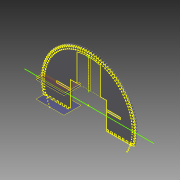
# Autodesk Inventor part: Spur Gear2
Saved by Autodesk Inventor 2013 (Build 170138000, 138)
## iProperties
Created: 2013-02-22
Part Number: Spur Gear2
Material: Steel
Document SubType Name: Modeling
Designer: Nano
Categories: <?xml version="1.0" encoding="UTF-16"?> <MemberInstance><Categories><FamilyTemplate><FamilyTemplateParameter ValueType="xs:double" Id="1" ObjectReferenceKey="da_z" ObjectType="kUserParameterObject"/><FamilyTemplateParameter ValueType="xs:double" Id="2" ObjectReferenceKey="da_b" ObjectType="kUserParameterObject"/><FamilyTemplateParameter ValueType="xs:double" Id="3" ObjectReferenceKey="da_beta" ObjectType="kUserParameterObject"/><FamilyTemplateParameter ValueType="xs:double" Id="4" ObjectReferenceKey="da_da" ObjectType="kUserParameterObject"/><FamilyTemplateParameter ValueType="xs:double" Id="5" ObjectReferenceKey="da_aw" ObjectType="kUserParameterObject"/><FamilyTemplateParameter ValueType="xs:string" Id="6" ObjectReferenceKey="EAIAABAAAAC/AAAAAAAAAIAAAAAAAAAA" ObjectType="83910656" SubObjectId="SurfaceGeometry"/></FamilyTemplate><ParamToTemplateMap><ParamToTemplate CategoryParameter="//CategoryParameter[@InternalName='046C89C9-8512-4d59-83FE-43B91F4F132A']" TemplateParameter="1"/><ParamToTemplate CategoryParameter="//CategoryParameter[@InternalName='2552DF32-E462-4b46-AEBF-C6C7768E72AC']" TemplateParameter="2"/><ParamToTemplate CategoryParameter="//CategoryParameter[@InternalName='C9EE641D-15FC-4fae-A226-E94C4372FDD7']" TemplateParameter="3"/><ParamToTemplate><ParamToTemplate CategoryParameter="//CategoryParameter[@InternalName='00B6519A-459B-49c7-AD84-2E56D39A5744']" ConstantValue="0.000000"/></ParamToTemplate><ParamToTemplate><ParamToTemplate CategoryParameter="//CategoryParameter[@InternalName='04B31F0E-C7A6-4894-AA32-9629BEFACF47']" ConstantValue="1.000000"/></ParamToTemplate><ParamToTemplate><ParamToTemplate CategoryParameter="//CategoryParameter[@InternalName='43CBEC2E-7847-49e7-A936-2F7889FCB2D9']" ConstantValue="0.250000"/></ParamToTemplate><ParamToTemplate><ParamToTemplate CategoryParameter="//CategoryParameter[@InternalName='B1EFC894-105D-4ebd-86BF-FA20ED196853']" ConstantValue="0.350000"/></ParamToTemplate><ParamToTemplate><ParamToTemplate CategoryParameter="//CategoryParameter[@InternalName='51175063-3D10-4879-93E8-6246FE8B403D']" ConstantValue="2060110000.000000"/></ParamToTemplate><ParamToTemplate><ParamToTemplate CategoryParameter="//CategoryParameter[@InternalName='A3A52E27-4454-46a9-B0BD-C932399B70AF']" ConstantValue="0.300000"/></ParamToTemplate><ParamToTemplate><ParamToTemplate CategoryParameter="//CategoryParameter[@InternalName='91B76062-C214-41d9-B1B9-14D2AB99603D']" ConstantValue="0.254000"/></ParamToTemplate><ParamToTemplate><ParamToTemplate CategoryParameter="//CategoryParameter[@InternalName='374E806E-8B8A-4dda-A9AA-1039D6500AD2']" ConstantValue="3.937008"/></ParamToTemplate><ParamToTemplate><ParamToTemplate CategoryParameter="//CategoryParameter[@InternalName='2D373A89-B862-43d6-8D0B-0CBF12AB9F6C']" ConstantValue="0.349066"/></ParamToTemplate><ParamToTemplate CategoryParameter="//CategoryParameter[@InternalName='37777632-D6A2-4fac-9D53-DB8ACD95C989']" TemplateParameter="4"/><ParamToTemplate CategoryParameter="//CategoryParameter[@InternalName='FD1017F1-B727-4f7e-9707-0F86F1FF9423']" TemplateParameter="5"/><ParamToTemplate><ParamToTemplate CategoryParameter="//CategoryParameter[@InternalName='9E1B4470-B2D3-4ff1-B813-535BB4CDF51A']" ConstantValue="3520790.000000"/></ParamToTemplate><ParamToTemplate><ParamToTemplate CategoryParameter="//CategoryParameter[@InternalName='F8452263-BFF6-458c-9FB1-07C4B99E95CD']" ConstantValue="11389170.000000"/></ParamToTemplate><ParamToTemplate><ParamToTemplate CategoryParameter="//CategoryParameter[@InternalName='3E3BB259-FD49-497f-8171-6EBC954A3479']" ConstantValue="2.000000"/></ParamToTemplate><ParamToTemplate CategoryParameter="//CategoryParameter[@InternalName='27C3BAF2-7550-4e4b-AE2C-0DB134B7D9B7']" TemplateParameter="6"/></ParamToTemplateMap><Category DisplayName="Gear" InternalName="DC85795E-93AB-48d5-8EEE-5A27447B64BD" Mnemonic="Gear"><CategoryParameter DisplayName="z" InternalName="046C89C9-8512-4d59-83FE-43B91F4F132A" Mnemonic="z"/><CategoryParameter DisplayName="b" InternalName="2552DF32-E462-4b46-AEBF-C6C7768E72AC" Mnemonic="b"/><CategoryParameter DisplayName="||b|" InternalName="C9EE641D-15FC-4fae-A226-E94C4372FDD7" Mnemonic="beta"/><CategoryParameter DisplayName="x" InternalName="00B6519A-459B-49c7-AD84-2E56D39A5744" Mnemonic="x"/><CategoryParameter DisplayName="a*" InternalName="04B31F0E-C7A6-4894-AA32-9629BEFACF47" Mnemonic="a"/><CategoryParameter DisplayName="c*" InternalName="43CBEC2E-7847-49e7-A936-2F7889FCB2D9" Mnemonic="c"/><CategoryParameter DisplayName="r|.f|*" InternalName="B1EFC894-105D-4ebd-86BF-FA20ED196853" Mnemonic="rf"/><CategoryParameter DisplayName="E" InternalName="51175063-3D10-4879-93E8-6246FE8B403D" Mnemonic="E"/><CategoryParameter DisplayName="||m|" InternalName="A3A52E27-4454-46a9-B0BD-C932399B70AF" Mnemonic="mi"/><Category DisplayName="SpurGear" InternalName="26C5A22E-A91E-4dfd-A3B3-23CCAFAE1764" Mnemonic="SpurGear"><CategoryParameter DisplayName="m" InternalName="91B76062-C214-41d9-B1B9-14D2AB99603D" Mnemonic="m"/><CategoryParameter DisplayName="P" InternalName="374E806E-8B8A-4dda-A9AA-1039D6500AD2" Mnemonic="PP"/><CategoryParameter DisplayName="||a|" InternalName="2D373A89-B862-43d6-8D0B-0CBF12AB9F6C" Mnemonic="alpha"/><CategoryParameter DisplayName="d|.a|" InternalName="37777632-D6A2-4fac-9D53-DB8ACD95C989" Mnemonic="da"/><CategoryParameter DisplayName="a|.w|" InternalName="FD1017F1-B727-4f7e-9707-0F86F1FF9423" Mnemonic="aw"/><CategoryParameter DisplayName="||s||.Flim|" InternalName="9E1B4470-B2D3-4ff1-B813-535BB4CDF51A" Mnemonic="sFlim"/><CategoryParameter DisplayName="||s||.Hlim|" InternalName="F8452263-BFF6-458c-9FB1-07C4B99E95CD" Mnemonic="sHlim"/><CategoryParameter DisplayName="type" InternalName="3E3BB259-FD49-497f-8171-6EBC954A3479" Mnemonic="type"/><CategoryParameter DisplayName="PitchDiameter" InternalName="27C3BAF2-7550-4e4b-AE2C-0DB134B7D9B7" Mnemonic="IDS_PITCHDIAM"/></Category></Category></Categories></MemberInstance>
Density: 1 g/cm^3
CustomPartVersion: 1
Author: Nano
Autodesk Inventor part; units mm, degrees
(part 1 of 2)
ref_plane "YZ Plane" through (0, 0, 0) normal (1, 0, 0) x (0, 1, 0)
ref_plane "XZ Plane" through (0, 0, 0) normal (0, 1, 0) x (-1, 0, 0)
ref_plane "XY Plane" through (0, 0, 0) normal (0, 0, 1) x (1, 0, 0)
sketch "Sketch1" plane through (0, 0, 0) normal (0, 0, 1) x (1, 0, 0)
  circle A0 centre (0, 0) radius 154.94
  dimension "d0" = 309.88
  constraints: 1 centre point
  measures "d0" diameter of A0
extrude "Extrusion1" add sketch "Sketch1" along normal blind 6.35
sketch "Sketch2" plane through (0, 0, 0) normal (0, 0, -1) x (-1, 0, 0)
  circle A0 centre (0, 0) radius 154.94 projected
  circle A1 centre (0, 0) radius 152.4
  dimension "d3" = 304.8
  constraints: 1 centre point, 1 coincident
  measures "d3" diameter of A1
surface extrude "Pitch Diameter" sketch "Sketch2" against normal through all shown no curves A1
ref_plane "Work Plane1" through (0, 0, 0) normal (1, 0, 0) x (0, 1, 0)
ref_plane "Work Plane2" through (0, 0, 0) normal (0.9996573, 0.0261769, 0) x (0, 0, 1)
ref_plane "Work Plane3" through (0, 0, 3.175) normal (0, 0, -1) x (-1, 0, 0)
spur gear teeth "Spur Gear" teeth 120 pitch diameter 304.8 tip diameter 309.88 root diameter 298.45 face width 6.35 start plane through (0, 0, 0) normal (0, 0, -1) x (-1, 0, 0)
sketch "Sketch3" plane through (0, 0, 6.35) normal (0, 0, 1) x (1, 0, 0)
  line L0 (-226.2292, -43.1165) -> (223.5893, -43.1165)
  constraints: 2 end point
split body "Split1" sketch "Sketch3" result one side removed curves L0 removed pieces at (21.5954, -83.6344, 0.5)
sketch "Sketch4" plane through (0, 0, 6.35) normal (0, 0, 1) x (1, 0, 0)
  line L0 (-142.8603, -43.1165) -> (142.8603, -43.1165) projected
  line L1 (-59.5312, -44.45) -> (59.5312, -44.45)
  line L2 (59.5312, -44.45) -> (59.5312, 44.45)
  line L3 (59.5312, 44.45) -> (38.1, 44.45)
  line L4 (-59.5312, 44.45) -> (-59.5312, -44.45)
  line L5 (-59.5312, -44.45) -> (59.5312, 44.45) construction
  line L6 (59.5312, -44.45) -> (-59.5312, 44.45) construction
  line L7 (-38.1, -3.175) -> (38.1, -3.175)
  line L8 (38.1, -3.175) -> (38.1, 133.985)
  line L9 (38.1, 133.985) -> (-38.1, 133.985)
  line L10 (-38.1, 133.985) -> (-38.1, -3.175)
  line L11 (-38.1, -3.175) -> (38.1, 133.985) construction
  line L12 (38.1, -3.175) -> (-38.1, 133.985) construction
  arc A0 (-133.0152, -43.1165) -> (38.1, 133.985) centre (0, -0.4192) ccw
  arc A1 (-38.1, 133.985) -> (-133.0152, -43.1165) centre (0, -0.4192) ccw
  arc A2 (38.1, 133.985) -> (-38.1, 133.985) centre (0, -0.4192) ccw
  line L13 (-38.1, 44.45) -> (-59.5312, 44.45)
  line L14 (38.1, 44.45) -> (-38.1, 44.45)
  point P0 (0, 0)
  point P1 (0, 65.405)
  dimension "d20" = 119.0625
  dimension "d21" = 88.9
  dimension "d22" = 76.2
  dimension "d23" = 137.16
  dimension "d24" = 279.4
  constraints: 28 end point, 6 parallel, 6 point on circle, 4 midpoint, 3 centre point, 3 point on line, 2 perpendicular
  measures "d20" distance of L1.start L1.end
  measures "d21" distance of L2.end L1.end
  measures "d22" distance of L7.start L7.end
  measures "d23" distance of L8.end L7.end
  measures "d24" diameter of A0
extrude "Extrusion2" cut sketch "Sketch4" against normal through all contours L4 L13 L10 L7 L8 L3 L2 L0 | L0 L2 L1 L4 | A2 L9 | L9 L8 L14 L10 | L14 L8 L7 L10
ref_plane "Work Plane4" through (-93.1308, -43.1165, 3.175) normal (0, -1, 0) x (1, 0, 0)
sketch "Sketch5" plane through (-93.1308, -43.1165, 3.175) normal (0, -1, 0) x (1, 0, 0)
  line L0 (-36.2504, 3.175) -> (-36.2504, -3.175) projected
  line L1 (-36.2504, -3.175) -> (-42.6004, -3.175) projected
  line L2 (-42.6004, -3.175) -> (-42.6004, 3.175) projected
  line L3 (-42.6004, 3.175) -> (-36.2504, 3.175) projected
  line L4 (-23.5504, 3.175) -> (-23.5504, -3.175) projected
  line L5 (-23.5504, -3.175) -> (-29.9004, -3.175) projected
  line L6 (-29.9004, -3.175) -> (-29.9004, 3.175) projected
  line L7 (-29.9004, 3.175) -> (-23.5504, 3.175) projected
  line L8 (-10.8504, 3.175) -> (-10.8504, -3.175) projected
  line L9 (-10.8504, -3.175) -> (-17.2004, -3.175) projected
  line L10 (-17.2004, -3.175) -> (-17.2004, 3.175) projected
  line L11 (-17.2004, 3.175) -> (-10.8504, 3.175) projected
  line L12 (1.8496, 3.175) -> (1.8496, -3.175) projected
  line L13 (1.8496, -3.175) -> (-4.5004, -3.175) projected
  line L14 (-4.5004, -3.175) -> (-4.5004, 3.175) projected
  line L15 (-4.5004, 3.175) -> (1.8496, 3.175) projected
  line L16 (14.5496, 3.175) -> (14.5496, -3.175) projected
  line L17 (14.5496, -3.175) -> (8.1996, -3.175) projected
  line L18 (8.1996, -3.175) -> (8.1996, 3.175) projected
  line L19 (8.1996, 3.175) -> (14.5496, 3.175) projected
  line L20 (27.2496, 3.175) -> (27.2496, -3.175) projected
  line L21 (27.2496, -3.175) -> (20.8996, -3.175) projected
  line L22 (20.8996, -3.175) -> (20.8996, 3.175) projected
  line L23 (20.8996, 3.175) -> (27.2496, 3.175) projected
  line L24 (-49.7295, -3.175) -> (33.5996, -25.4) projected
  line L25 (33.5996, -25.4) -> (33.5996, 25.4) projected
  line L26 (33.5996, 25.4) -> (-49.7295, 3.175) projected
  line L27 (-49.7295, 3.175) -> (-49.7295, -3.175) projected
  point P0 (93.1308, -3.175)
extrude "Extrusion3" cut sketch "Sketch5" against normal blind 6.35
sketch "Sketch6" plane through (0, 0, 6.35) normal (0, 0, 1) x (1, 0, 0)
  line L0 (-65.8813, -36.7665) -> (-59.5312, -36.7665) projected
  line L1 (-59.5312, -36.7665) -> (-59.5312, 44.45) projected
  line L2 (-59.5312, 44.45) -> (-38.1, 44.45) projected
  line L3 (-38.1, 44.45) -> (-38.1, 133.985) projected
  arc A0 (38.1, 133.985) -> (-38.1, 133.985) centre (0, -0.4192) ccw projected
  line L4 (38.1, 133.985) -> (38.1, 44.45) projected
  line L5 (38.1, 44.45) -> (59.5312, 44.45) projected
  line L6 (59.5312, 44.45) -> (59.5312, -43.1165) projected
  line L7 (59.5312, -43.1165) -> (142.8603, -43.1165) projected
  arc A1 (142.8603, -43.1165) -> (143.3542, -41.4448) centre (0, 0) ccw projected
  arc A2 (143.3542, -41.4448) -> (149.3949, -41.0801) centre (144.1598, -4.5833) ccw projected
  arc A3 (149.3949, -41.0801) -> (149.9198, -39.121) centre (0, 0) ccw projected
  arc A4 (149.9198, -39.121) -> (144.8708, -35.7848) centre (127.1377, -68.1106) ccw projected
  arc A5 (144.8708, -35.7848) -> (145.3268, -33.8855) centre (0, 0) ccw projected
  arc A6 (145.3268, -33.8855) -> (151.3401, -33.2051) centre (144.2021, 2.9677) ccw projected
  arc A7 (151.3401, -33.2051) -> (151.7618, -31.2212) centre (0, 0) ccw projected
  arc A8 (151.7618, -31.2212) -> (146.5451, -28.1538) centre (130.5281, -61.3634) ccw projected
  arc A9 (146.5451, -28.1538) -> (146.9011, -26.2332) centre (0, 0) ccw projected
  arc A10 (146.9011, -26.2332) -> (152.8705, -25.239) centre (143.8491, 10.5106) ccw projected
  arc A11 (152.8705, -25.239) -> (153.1878, -23.2358) centre (0, 0) ccw projected
  arc A12 (153.1878, -23.2358) -> (147.8177, -20.4457) centre (133.5607, -54.448) ccw projected
  arc A13 (147.8177, -20.4457) -> (148.0727, -18.509) centre (0, 0) ccw projected
  arc A14 (148.0727, -18.509) -> (153.9819, -17.2038) centre (143.1019, 18.0247) ccw projected
  arc A15 (153.9819, -17.2038) -> (154.1939, -15.1868) centre (0, 0) ccw projected
  arc A16 (154.1939, -15.1868) -> (148.6852, -12.6815) centre (136.2272, -47.3834) ccw projected
  arc A17 (148.6852, -12.6815) -> (148.8384, -10.7342) centre (0, 0) ccw projected
  arc A18 (148.8384, -10.7342) -> (154.6713, -9.1214) centre (141.9624, 25.4894) ccw projected
  arc A19 (154.6713, -9.1214) -> (154.7774, -7.0961) centre (0, 0) ccw projected
  arc A20 (154.7774, -7.0961) -> (149.1451, -4.8825) centre (138.5204, -40.1889) ccw projected
  arc A21 (149.1451, -4.8825) -> (149.1962, -2.9298) centre (0, 0) ccw projected
  arc A22 (149.1962, -2.9298) -> (154.9367, -1.0141) centre (140.4339, 32.8842) ccw projected
  arc A23 (154.9367, -1.0141) -> (154.9367, 1.0141) centre (0, 0) ccw projected
  arc A24 (154.9367, 1.0141) -> (149.1962, 2.9298) centre (140.4339, -32.8842) ccw projected
  arc A25 (149.1962, 2.9298) -> (149.1451, 4.8825) centre (0, 0) ccw projected
  arc A26 (149.1451, 4.8825) -> (154.7774, 7.0961) centre (138.5204, 40.1889) ccw projected
  arc A27 (154.7774, 7.0961) -> (154.6713, 9.1214) centre (0, 0) ccw projected
  arc A28 (154.6713, 9.1214) -> (148.8384, 10.7342) centre (141.9624, -25.4894) ccw projected
  arc A29 (148.8384, 10.7342) -> (148.6852, 12.6815) centre (0, 0) ccw projected
  arc A30 (148.6852, 12.6815) -> (154.1939, 15.1868) centre (136.2272, 47.3834) ccw projected
  arc A31 (154.1939, 15.1868) -> (153.9819, 17.2038) centre (0, 0) ccw projected
  arc A32 (153.9819, 17.2038) -> (148.0727, 18.509) centre (143.1019, -18.0247) ccw projected
  arc A33 (148.0727, 18.509) -> (147.8177, 20.4457) centre (0, 0) ccw projected
  arc A34 (147.8177, 20.4457) -> (153.1878, 23.2358) centre (133.5607, 54.448) ccw projected
  arc A35 (153.1878, 23.2358) -> (152.8705, 25.239) centre (0, 0) ccw projected
  arc A36 (152.8705, 25.239) -> (146.9011, 26.2332) centre (143.8491, -10.5106) ccw projected
  arc A37 (146.9011, 26.2332) -> (146.5451, 28.1538) centre (0, 0) ccw projected
  arc A38 (146.5451, 28.1538) -> (151.7618, 31.2212) centre (130.5281, 61.3634) ccw projected
  arc A39 (151.7618, 31.2212) -> (151.3401, 33.2051) centre (0, 0) ccw projected
  arc A40 (151.3401, 33.2051) -> (145.3268, 33.8855) centre (144.2021, -2.9677) ccw projected
  arc A41 (145.3268, 33.8855) -> (144.8708, 35.7848) centre (0, 0) ccw projected
  arc A42 (144.8708, 35.7848) -> (149.9198, 39.121) centre (127.1377, 68.1106) ccw projected
  arc A43 (149.9198, 39.121) -> (149.3949, 41.0801) centre (0, 0) ccw projected
  arc A44 (149.3949, 41.0801) -> (143.3542, 41.4448) centre (144.1598, 4.5833) ccw projected
  arc A45 (143.3542, 41.4448) -> (142.7994, 43.3177) centre (0, 0) ccw projected
  arc A46 (142.7994, 43.3177) -> (147.6669, 46.9136) centre (123.3988, 74.6712) ccw projected
  arc A47 (147.6669, 46.9136) -> (147.0402, 48.8425) centre (0, 0) ccw projected
  arc A48 (147.0402, 48.8425) -> (140.9887, 48.8906) centre (143.7223, 12.1217) ccw projected
  arc A49 (140.9887, 48.8906) -> (140.3366, 50.7319) centre (0, 0) ccw projected
  arc A50 (140.3366, 50.7319) -> (145.0093, 54.5776) centre (119.3217, 81.027) ccw projected
  arc A51 (145.0093, 54.5776) -> (144.2824, 56.4711) centre (0, 0) ccw projected
  arc A52 (144.2824, 56.4711) -> (138.2367, 56.2024) centre (142.891, 19.627) ccw projected
  arc A53 (138.2367, 56.2024) -> (137.4892, 58.007) centre (0, 0) ccw projected
  arc A54 (137.4892, 58.007) -> (141.9542, 62.092) centre (114.9175, 87.1608) ccw projected
  arc A55 (141.9542, 62.092) -> (141.1292, 63.9448) centre (0, 0) ccw projected
  arc A56 (141.1292, 63.9448) -> (135.1059, 63.3601) centre (141.6679, 27.0784) ccw projected
  arc A57 (135.1059, 63.3601) -> (134.2649, 65.1232) centre (0, 0) ccw projected
  arc A58 (134.2649, 65.1232) -> (138.51, 69.4362) centre (110.1984, 93.0557) ccw projected
  arc A59 (138.51, 69.4362) -> (137.5892, 71.2433) centre (0, 0) ccw projected
  arc A60 (137.5892, 71.2433) -> (131.6047, 70.3442) centre (140.0566, 34.4556) ccw projected
  arc A61 (131.6047, 70.3442) -> (130.6726, 72.0608) centre (0, 0) ccw projected
  arc A62 (130.6726, 72.0608) -> (134.6861, 76.5901) centre (105.1772, 98.6955) ccw projected
  arc A63 (134.6861, 76.5901) -> (133.6721, 78.3466) centre (0, 0) ccw projected
  arc A64 (133.6721, 78.3466) -> (127.7428, 77.1354) centre (138.0614, 41.7384) ccw projected
  arc A65 (127.7428, 77.1354) -> (126.7222, 78.8009) centre (0, 0) ccw projected
  arc A66 (126.7222, 78.8009) -> (130.4931, 83.5341) centre (99.8678, 104.0648) ccw projected
  arc A67 (130.4931, 83.5341) -> (129.3885, 85.235) centre (0, 0) ccw projected
  arc A68 (129.3885, 85.235) -> (123.5308, 83.7153) centre (135.6878, 48.9068) ccw projected
  arc A69 (123.5308, 83.7153) -> (122.4244, 85.3251) centre (0, 0) ccw projected
  arc A70 (122.4244, 85.3251) -> (125.9425, 90.2491) centre (94.2846, 109.1488) ccw projected
  arc A71 (125.9425, 90.2491) -> (124.7504, 91.8899) centre (0, 0) ccw projected
  arc A72 (124.7504, 91.8899) -> (118.9802, 90.0656) centre (132.9422, 55.9411) ccw projected
  arc A73 (118.9802, 90.0656) -> (117.7911, 91.6153) centre (0, 0) ccw projected
  arc A74 (117.7911, 91.6153) -> (121.0466, 96.7167) centre (88.4429, 113.9337) ccw projected
  arc A75 (121.0466, 96.7167) -> (119.7702, 98.2929) centre (0, 0) ccw projected
  arc A76 (119.7702, 98.2929) -> (114.1034, 96.1691) centre (129.8323, 62.8221) ccw projected
  arc A77 (114.1034, 96.1691) -> (112.8349, 97.6545) centre (0, 0) ccw projected
  arc A78 (112.8349, 97.6545) -> (115.8189, 102.9193) centre (82.3589, 118.4063) ccw projected
  arc A79 (115.8189, 102.9193) -> (114.4618, 104.4265) centre (0, 0) ccw projected
  arc A80 (114.4618, 104.4265) -> (108.914, 102.0091) centre (126.3665, 69.5309) ccw projected
  arc A81 (108.914, 102.0091) -> (107.5694, 103.426) centre (0, 0) ccw projected
  arc A82 (107.5694, 103.426) -> (110.2738, 108.8397) centre (76.0491, 122.5544) ccw projected
  arc A83 (110.2738, 108.8397) -> (108.8397, 110.2738) centre (0, 0) ccw projected
  arc A84 (108.8397, 110.2738) -> (103.426, 107.5694) centre (122.5544, 76.0491) ccw projected
  arc A85 (103.426, 107.5694) -> (102.0091, 108.914) centre (0, 0) ccw projected
  arc A86 (102.0091, 108.914) -> (104.4265, 114.4618) centre (69.5309, 126.3665) ccw projected
  arc A87 (104.4265, 114.4618) -> (102.9193, 115.8189) centre (0, 0) ccw projected
  arc A88 (102.9193, 115.8189) -> (97.6545, 112.8349) centre (118.4063, 82.3589) ccw projected
  arc A89 (97.6545, 112.8349) -> (96.1691, 114.1034) centre (0, 0) ccw projected
  arc A90 (96.1691, 114.1034) -> (98.2929, 119.7702) centre (62.8221, 129.8323) ccw projected
  arc A91 (98.2929, 119.7702) -> (96.7167, 121.0466) centre (0, 0) ccw projected
  arc A92 (96.7167, 121.0466) -> (91.6153, 117.7911) centre (113.9337, 88.4429) ccw projected
  arc A93 (91.6153, 117.7911) -> (90.0656, 118.9802) centre (0, 0) ccw projected
  arc A94 (90.0656, 118.9802) -> (91.8899, 124.7504) centre (55.9411, 132.9422) ccw projected
  arc A95 (91.8899, 124.7504) -> (90.2491, 125.9425) centre (0, 0) ccw projected
  arc A96 (90.2491, 125.9425) -> (85.3251, 122.4244) centre (109.1488, 94.2846) ccw projected
  arc A97 (85.3251, 122.4244) -> (83.7153, 123.5308) centre (0, 0) ccw projected
  arc A98 (83.7153, 123.5308) -> (85.235, 129.3885) centre (48.9068, 135.6878) ccw projected
  arc A99 (85.235, 129.3885) -> (83.5341, 130.4931) centre (0, 0) ccw projected
  arc A100 (83.5341, 130.4931) -> (78.8009, 126.7222) centre (104.0648, 99.8678) ccw projected
  arc A101 (78.8009, 126.7222) -> (77.1354, 127.7428) centre (0, 0) ccw projected
  arc A102 (77.1354, 127.7428) -> (78.3466, 133.6721) centre (41.7384, 138.0614) ccw projected
  arc A103 (78.3466, 133.6721) -> (76.5901, 134.6861) centre (0, 0) ccw projected
  arc A104 (76.5901, 134.6861) -> (72.0608, 130.6726) centre (98.6955, 105.1772) ccw projected
  arc A105 (72.0608, 130.6726) -> (70.3442, 131.6047) centre (0, 0) ccw projected
  arc A106 (70.3442, 131.6047) -> (71.2433, 137.5892) centre (34.4556, 140.0566) ccw projected
  arc A107 (71.2433, 137.5892) -> (69.4362, 138.51) centre (0, 0) ccw projected
  arc A108 (69.4362, 138.51) -> (65.1232, 134.2649) centre (93.0557, 110.1984) ccw projected
  arc A109 (65.1232, 134.2649) -> (63.3601, 135.1059) centre (0, 0) ccw projected
  arc A110 (63.3601, 135.1059) -> (63.9448, 141.1292) centre (27.0784, 141.6679) ccw projected
  arc A111 (63.9448, 141.1292) -> (62.092, 141.9542) centre (0, 0) ccw projected
  arc A112 (62.092, 141.9542) -> (58.007, 137.4892) centre (87.1608, 114.9175) ccw projected
  arc A113 (58.007, 137.4892) -> (56.2024, 138.2367) centre (0, 0) ccw projected
  arc A114 (56.2024, 138.2367) -> (56.4711, 144.2824) centre (19.627, 142.891) ccw projected
  arc A115 (56.4711, 144.2824) -> (54.5776, 145.0093) centre (0, 0) ccw projected
  arc A116 (54.5776, 145.0093) -> (50.7319, 140.3366) centre (81.027, 119.3217) ccw projected
  arc A117 (50.7319, 140.3366) -> (48.8906, 140.9887) centre (0, 0) ccw projected
  arc A118 (48.8906, 140.9887) -> (48.8425, 147.0402) centre (12.1217, 143.7223) ccw projected
  arc A119 (48.8425, 147.0402) -> (46.9136, 147.6669) centre (0, 0) ccw projected
  arc A120 (46.9136, 147.6669) -> (43.3177, 142.7994) centre (74.6712, 123.3988) ccw projected
  arc A121 (43.3177, 142.7994) -> (41.4448, 143.3542) centre (0, 0) ccw projected
  arc A122 (41.4448, 143.3542) -> (41.0801, 149.3949) centre (4.5833, 144.1598) ccw projected
  arc A123 (41.0801, 149.3949) -> (39.121, 149.9198) centre (0, 0) ccw projected
  arc A124 (39.121, 149.9198) -> (35.7848, 144.8708) centre (68.1106, 127.1377) ccw projected
  arc A125 (35.7848, 144.8708) -> (33.8855, 145.3268) centre (0, 0) ccw projected
  arc A126 (33.8855, 145.3268) -> (33.2051, 151.3401) centre (-2.9677, 144.2021) ccw projected
  arc A127 (33.2051, 151.3401) -> (31.2212, 151.7618) centre (0, 0) ccw projected
  arc A128 (31.2212, 151.7618) -> (28.1538, 146.5451) centre (61.3634, 130.5281) ccw projected
  arc A129 (28.1538, 146.5451) -> (26.2332, 146.9011) centre (0, 0) ccw projected
  arc A130 (26.2332, 146.9011) -> (25.239, 152.8705) centre (-10.5106, 143.8491) ccw projected
  arc A131 (25.239, 152.8705) -> (23.2358, 153.1878) centre (0, 0) ccw projected
  arc A132 (23.2358, 153.1878) -> (20.4457, 147.8177) centre (54.448, 133.5607) ccw projected
  arc A133 (20.4457, 147.8177) -> (18.509, 148.0727) centre (0, 0) ccw projected
  arc A134 (18.509, 148.0727) -> (17.2038, 153.9819) centre (-18.0247, 143.1019) ccw projected
  arc A135 (17.2038, 153.9819) -> (15.1868, 154.1939) centre (0, 0) ccw projected
  arc A136 (15.1868, 154.1939) -> (12.6815, 148.6852) centre (47.3834, 136.2272) ccw projected
  arc A137 (12.6815, 148.6852) -> (10.7342, 148.8384) centre (0, 0) ccw projected
  arc A138 (10.7342, 148.8384) -> (9.1214, 154.6713) centre (-25.4894, 141.9624) ccw projected
  arc A139 (9.1214, 154.6713) -> (7.0961, 154.7774) centre (0, 0) ccw projected
  arc A140 (7.0961, 154.7774) -> (4.8825, 149.1451) centre (40.1889, 138.5204) ccw projected
  arc A141 (4.8825, 149.1451) -> (2.9298, 149.1962) centre (0, 0) ccw projected
  arc A142 (2.9298, 149.1962) -> (1.0141, 154.9367) centre (-32.8842, 140.4339) ccw projected
  arc A143 (1.0141, 154.9367) -> (-1.0141, 154.9367) centre (0, 0) ccw projected
  arc A144 (-1.0141, 154.9367) -> (-2.9298, 149.1962) centre (32.8842, 140.4339) ccw projected
  arc A145 (-2.9298, 149.1962) -> (-4.8825, 149.1451) centre (0, 0) ccw projected
  arc A146 (-4.8825, 149.1451) -> (-7.0961, 154.7774) centre (-40.1889, 138.5204) ccw projected
  arc A147 (-7.0961, 154.7774) -> (-9.1214, 154.6713) centre (0, 0) ccw projected
  arc A148 (-9.1214, 154.6713) -> (-10.7342, 148.8384) centre (25.4894, 141.9624) ccw projected
  arc A149 (-10.7342, 148.8384) -> (-12.6815, 148.6852) centre (0, 0) ccw projected
  arc A150 (-12.6815, 148.6852) -> (-15.1868, 154.1939) centre (-47.3834, 136.2272) ccw projected
  arc A151 (-15.1868, 154.1939) -> (-17.2038, 153.9819) centre (0, 0) ccw projected
  arc A152 (-17.2038, 153.9819) -> (-18.509, 148.0727) centre (18.0247, 143.1019) ccw projected
  arc A153 (-18.509, 148.0727) -> (-20.4457, 147.8177) centre (0, 0) ccw projected
  arc A154 (-20.4457, 147.8177) -> (-23.2358, 153.1878) centre (-54.448, 133.5607) ccw projected
  arc A155 (-23.2358, 153.1878) -> (-25.239, 152.8705) centre (0, 0) ccw projected
  arc A156 (-25.239, 152.8705) -> (-26.2332, 146.9011) centre (10.5106, 143.8491) ccw projected
  arc A157 (-26.2332, 146.9011) -> (-28.1538, 146.5451) centre (0, 0) ccw projected
  arc A158 (-28.1538, 146.5451) -> (-31.2212, 151.7618) centre (-61.3634, 130.5281) ccw projected
  arc A159 (-31.2212, 151.7618) -> (-33.2051, 151.3401) centre (0, 0) ccw projected
  arc A160 (-33.2051, 151.3401) -> (-33.8855, 145.3268) centre (2.9677, 144.2021) ccw projected
  arc A161 (-33.8855, 145.3268) -> (-35.7848, 144.8708) centre (0, 0) ccw projected
  arc A162 (-35.7848, 144.8708) -> (-39.121, 149.9198) centre (-68.1106, 127.1377) ccw projected
  arc A163 (-39.121, 149.9198) -> (-41.0801, 149.3949) centre (0, 0) ccw projected
  arc A164 (-41.0801, 149.3949) -> (-41.4448, 143.3542) centre (-4.5833, 144.1598) ccw projected
  arc A165 (-41.4448, 143.3542) -> (-43.3177, 142.7994) centre (0, 0) ccw projected
  arc A166 (-43.3177, 142.7994) -> (-46.9136, 147.6669) centre (-74.6712, 123.3988) ccw projected
  arc A167 (-46.9136, 147.6669) -> (-48.8425, 147.0402) centre (0, 0) ccw projected
  arc A168 (-48.8425, 147.0402) -> (-48.8906, 140.9887) centre (-12.1217, 143.7223) ccw projected
  arc A169 (-48.8906, 140.9887) -> (-50.7319, 140.3366) centre (0, 0) ccw projected
  arc A170 (-50.7319, 140.3366) -> (-54.5776, 145.0093) centre (-81.027, 119.3217) ccw projected
  arc A171 (-54.5776, 145.0093) -> (-56.4711, 144.2824) centre (0, 0) ccw projected
  arc A172 (-56.4711, 144.2824) -> (-56.2024, 138.2367) centre (-19.627, 142.891) ccw projected
  arc A173 (-56.2024, 138.2367) -> (-58.007, 137.4892) centre (0, 0) ccw projected
  arc A174 (-58.007, 137.4892) -> (-62.092, 141.9542) centre (-87.1608, 114.9175) ccw projected
  arc A175 (-62.092, 141.9542) -> (-63.9448, 141.1292) centre (0, 0) ccw projected
  arc A176 (-63.9448, 141.1292) -> (-63.3601, 135.1059) centre (-27.0784, 141.6679) ccw projected
  arc A177 (-63.3601, 135.1059) -> (-65.1232, 134.2649) centre (0, 0) ccw projected
  arc A178 (-65.1232, 134.2649) -> (-69.4362, 138.51) centre (-93.0557, 110.1984) ccw projected
  arc A179 (-69.4362, 138.51) -> (-71.2433, 137.5892) centre (0, 0) ccw projected
  arc A180 (-71.2433, 137.5892) -> (-70.3442, 131.6047) centre (-34.4556, 140.0566) ccw projected
  arc A181 (-70.3442, 131.6047) -> (-72.0608, 130.6726) centre (0, 0) ccw projected
  arc A182 (-72.0608, 130.6726) -> (-76.5901, 134.6861) centre (-98.6955, 105.1772) ccw projected
  arc A183 (-76.5901, 134.6861) -> (-78.3466, 133.6721) centre (0, 0) ccw projected
  arc A184 (-78.3466, 133.6721) -> (-77.1354, 127.7428) centre (-41.7384, 138.0614) ccw projected
  arc A185 (-77.1354, 127.7428) -> (-78.8009, 126.7222) centre (0, 0) ccw projected
  arc A186 (-78.8009, 126.7222) -> (-83.5341, 130.4931) centre (-104.0648, 99.8678) ccw projected
  arc A187 (-83.5341, 130.4931) -> (-85.235, 129.3885) centre (0, 0) ccw projected
  arc A188 (-85.235, 129.3885) -> (-83.7153, 123.5308) centre (-48.9068, 135.6878) ccw projected
  arc A189 (-83.7153, 123.5308) -> (-85.3251, 122.4244) centre (0, 0) ccw projected
  arc A190 (-85.3251, 122.4244) -> (-90.2491, 125.9425) centre (-109.1488, 94.2846) ccw projected
  arc A191 (-90.2491, 125.9425) -> (-91.8899, 124.7504) centre (0, 0) ccw projected
  arc A192 (-91.8899, 124.7504) -> (-90.0656, 118.9802) centre (-55.9411, 132.9422) ccw projected
  arc A193 (-90.0656, 118.9802) -> (-91.6153, 117.7911) centre (0, 0) ccw projected
  arc A194 (-91.6153, 117.7911) -> (-96.7167, 121.0466) centre (-113.9337, 88.4429) ccw projected
  arc A195 (-96.7167, 121.0466) -> (-98.2929, 119.7702) centre (0, 0) ccw projected
  arc A196 (-98.2929, 119.7702) -> (-96.1691, 114.1034) centre (-62.8221, 129.8323) ccw projected
  arc A197 (-96.1691, 114.1034) -> (-97.6545, 112.8349) centre (0, 0) ccw projected
  arc A198 (-97.6545, 112.8349) -> (-102.9193, 115.8189) centre (-118.4063, 82.3589) ccw projected
  arc A199 (-102.9193, 115.8189) -> (-104.4265, 114.4618) centre (0, 0) ccw projected
  arc A200 (-104.4265, 114.4618) -> (-102.0091, 108.914) centre (-69.5309, 126.3665) ccw projected
  arc A201 (-102.0091, 108.914) -> (-103.426, 107.5694) centre (0, 0) ccw projected
  arc A202 (-103.426, 107.5694) -> (-108.8397, 110.2738) centre (-122.5544, 76.0491) ccw projected
  arc A203 (-108.8397, 110.2738) -> (-110.2738, 108.8397) centre (0, 0) ccw projected
  arc A204 (-110.2738, 108.8397) -> (-107.5694, 103.426) centre (-76.0491, 122.5544) ccw projected
  arc A205 (-107.5694, 103.426) -> (-108.914, 102.0091) centre (0, 0) ccw projected
  arc A206 (-108.914, 102.0091) -> (-114.4618, 104.4265) centre (-126.3665, 69.5309) ccw projected
  arc A207 (-114.4618, 104.4265) -> (-115.8189, 102.9193) centre (0, 0) ccw projected
  arc A208 (-115.8189, 102.9193) -> (-112.8349, 97.6545) centre (-82.3589, 118.4063) ccw projected
  arc A209 (-112.8349, 97.6545) -> (-114.1034, 96.1691) centre (0, 0) ccw projected
  arc A210 (-114.1034, 96.1691) -> (-119.7702, 98.2929) centre (-129.8323, 62.8221) ccw projected
  arc A211 (-119.7702, 98.2929) -> (-121.0466, 96.7167) centre (0, 0) ccw projected
  arc A212 (-121.0466, 96.7167) -> (-117.7911, 91.6153) centre (-88.4429, 113.9337) ccw projected
  arc A213 (-117.7911, 91.6153) -> (-118.9802, 90.0656) centre (0, 0) ccw projected
  arc A214 (-118.9802, 90.0656) -> (-124.7504, 91.8899) centre (-132.9422, 55.9411) ccw projected
  arc A215 (-124.7504, 91.8899) -> (-125.9425, 90.2491) centre (0, 0) ccw projected
  arc A216 (-125.9425, 90.2491) -> (-122.4244, 85.3251) centre (-94.2846, 109.1488) ccw projected
  arc A217 (-122.4244, 85.3251) -> (-123.5308, 83.7153) centre (0, 0) ccw projected
  arc A218 (-123.5308, 83.7153) -> (-129.3885, 85.235) centre (-135.6878, 48.9068) ccw projected
  arc A219 (-129.3885, 85.235) -> (-130.4931, 83.5341) centre (0, 0) ccw projected
  arc A220 (-130.4931, 83.5341) -> (-126.7222, 78.8009) centre (-99.8678, 104.0648) ccw projected
  arc A221 (-126.7222, 78.8009) -> (-127.7428, 77.1354) centre (0, 0) ccw projected
  arc A222 (-127.7428, 77.1354) -> (-133.6721, 78.3466) centre (-138.0614, 41.7384) ccw projected
  arc A223 (-133.6721, 78.3466) -> (-134.6861, 76.5901) centre (0, 0) ccw projected
  arc A224 (-134.6861, 76.5901) -> (-130.6726, 72.0608) centre (-105.1772, 98.6955) ccw projected
  arc A225 (-130.6726, 72.0608) -> (-131.6047, 70.3442) centre (0, 0) ccw projected
  arc A226 (-131.6047, 70.3442) -> (-137.5892, 71.2433) centre (-140.0566, 34.4556) ccw projected
  arc A227 (-137.5892, 71.2433) -> (-138.51, 69.4362) centre (0, 0) ccw projected
  arc A228 (-138.51, 69.4362) -> (-134.2649, 65.1232) centre (-110.1984, 93.0557) ccw projected
  arc A229 (-134.2649, 65.1232) -> (-135.1059, 63.3601) centre (0, 0) ccw projected
  arc A230 (-135.1059, 63.3601) -> (-141.1292, 63.9448) centre (-141.6679, 27.0784) ccw projected
  arc A231 (-141.1292, 63.9448) -> (-141.9542, 62.092) centre (0, 0) ccw projected
  arc A232 (-141.9542, 62.092) -> (-137.4892, 58.007) centre (-114.9175, 87.1608) ccw projected
  arc A233 (-137.4892, 58.007) -> (-138.2367, 56.2024) centre (0, 0) ccw projected
  arc A234 (-138.2367, 56.2024) -> (-144.2824, 56.4711) centre (-142.891, 19.627) ccw projected
  arc A235 (-144.2824, 56.4711) -> (-145.0093, 54.5776) centre (0, 0) ccw projected
  arc A236 (-145.0093, 54.5776) -> (-140.3366, 50.7319) centre (-119.3217, 81.027) ccw projected
  arc A237 (-140.3366, 50.7319) -> (-140.9887, 48.8906) centre (0, 0) ccw projected
  arc A238 (-140.9887, 48.8906) -> (-147.0402, 48.8425) centre (-143.7223, 12.1217) ccw projected
  arc A239 (-147.0402, 48.8425) -> (-147.6669, 46.9136) centre (0, 0) ccw projected
  arc A240 (-147.6669, 46.9136) -> (-142.7994, 43.3177) centre (-123.3988, 74.6712) ccw projected
  arc A241 (-142.7994, 43.3177) -> (-143.3542, 41.4448) centre (0, 0) ccw projected
  arc A242 (-143.3542, 41.4448) -> (-149.3949, 41.0801) centre (-144.1598, 4.5833) ccw projected
  arc A243 (-149.3949, 41.0801) -> (-149.9198, 39.121) centre (0, 0) ccw projected
  arc A244 (-149.9198, 39.121) -> (-144.8708, 35.7848) centre (-127.1377, 68.1106) ccw projected
  arc A245 (-144.8708, 35.7848) -> (-145.3268, 33.8855) centre (0, 0) ccw projected
  arc A246 (-145.3268, 33.8855) -> (-151.3401, 33.2051) centre (-144.2021, -2.9677) ccw projected
  arc A247 (-151.3401, 33.2051) -> (-151.7618, 31.2212) centre (0, 0) ccw projected
  arc A248 (-151.7618, 31.2212) -> (-146.5451, 28.1538) centre (-130.5281, 61.3634) ccw projected
  arc A249 (-146.5451, 28.1538) -> (-146.9011, 26.2332) centre (0, 0) ccw projected
  arc A250 (-146.9011, 26.2332) -> (-152.8705, 25.239) centre (-143.8491, -10.5106) ccw projected
  arc A251 (-152.8705, 25.239) -> (-153.1878, 23.2358) centre (0, 0) ccw projected
  arc A252 (-153.1878, 23.2358) -> (-147.8177, 20.4457) centre (-133.5607, 54.448) ccw projected
  arc A253 (-147.8177, 20.4457) -> (-148.0727, 18.509) centre (0, 0) ccw projected
  arc A254 (-148.0727, 18.509) -> (-153.9819, 17.2038) centre (-143.1019, -18.0247) ccw projected
  arc A255 (-153.9819, 17.2038) -> (-154.1939, 15.1868) centre (0, 0) ccw projected
  arc A256 (-154.1939, 15.1868) -> (-148.6852, 12.6815) centre (-136.2272, 47.3834) ccw projected
  arc A257 (-148.6852, 12.6815) -> (-148.8384, 10.7342) centre (0, 0) ccw projected
  arc A258 (-148.8384, 10.7342) -> (-154.6713, 9.1214) centre (-141.9624, -25.4894) ccw projected
  arc A259 (-154.6713, 9.1214) -> (-154.7774, 7.0961) centre (0, 0) ccw projected
  arc A260 (-154.7774, 7.0961) -> (-149.1451, 4.8825) centre (-138.5204, 40.1889) ccw projected
  arc A261 (-149.1451, 4.8825) -> (-149.1962, 2.9298) centre (0, 0) ccw projected
  arc A262 (-149.1962, 2.9298) -> (-154.9367, 1.0141) centre (-140.4339, -32.8842) ccw projected
  arc A263 (-154.9367, 1.0141) -> (-154.9367, -1.0141) centre (0, 0) ccw projected
  arc A264 (-154.9367, -1.0141) -> (-149.1962, -2.9298) centre (-140.4339, 32.8842) ccw projected
  arc A265 (-149.1962, -2.9298) -> (-149.1451, -4.8825) centre (0, 0) ccw projected
  arc A266 (-149.1451, -4.8825) -> (-154.7774, -7.0961) centre (-138.5204, -40.1889) ccw projected
  arc A267 (-154.7774, -7.0961) -> (-154.6713, -9.1214) centre (0, 0) ccw projected
  arc A268 (-154.6713, -9.1214) -> (-148.8384, -10.7342) centre (-141.9624, 25.4894) ccw projected
  arc A269 (-148.8384, -10.7342) -> (-148.6852, -12.6815) centre (0, 0) ccw projected
  arc A270 (-148.6852, -12.6815) -> (-154.1939, -15.1868) centre (-136.2272, -47.3834) ccw projected
  arc A271 (-154.1939, -15.1868) -> (-153.9819, -17.2038) centre (0, 0) ccw projected
  arc A272 (-153.9819, -17.2038) -> (-148.0727, -18.509) centre (-143.1019, 18.0247) ccw projected
  arc A273 (-148.0727, -18.509) -> (-147.8177, -20.4457) centre (0, 0) ccw projected
  arc A274 (-147.8177, -20.4457) -> (-153.1878, -23.2358) centre (-133.5607, -54.448) ccw projected
  arc A275 (-153.1878, -23.2358) -> (-152.8705, -25.239) centre (0, 0) ccw projected
  arc A276 (-152.8705, -25.239) -> (-146.9011, -26.2332) centre (-143.8491, 10.5106) ccw projected
  arc A277 (-146.9011, -26.2332) -> (-146.5451, -28.1538) centre (0, 0) ccw projected
  arc A278 (-146.5451, -28.1538) -> (-151.7618, -31.2212) centre (-130.5281, -61.3634) ccw projected
  arc A279 (-151.7618, -31.2212) -> (-151.3401, -33.2051) centre (0, 0) ccw projected
  arc A280 (-151.3401, -33.2051) -> (-145.3268, -33.8855) centre (-144.2021, 2.9677) ccw projected
  arc A281 (-145.3268, -33.8855) -> (-144.8708, -35.7848) centre (0, 0) ccw projected
  arc A282 (-144.8708, -35.7848) -> (-149.9198, -39.121) centre (-127.1377, -68.1106) ccw projected
  arc A283 (-149.9198, -39.121) -> (-149.3949, -41.0801) centre (0, 0) ccw projected
  arc A284 (-149.3949, -41.0801) -> (-143.3542, -41.4448) centre (-144.1598, -4.5833) ccw projected
  arc A285 (-143.3542, -41.4448) -> (-142.8603, -43.1165) centre (0, 0) ccw projected
  line L8 (-142.8603, -43.1165) -> (-142.8603, -36.7665) projected
  line L9 (-142.8603, -36.7665) -> (-135.7313, -36.7665) projected
  line L10 (-135.7313, -36.7665) -> (-135.7313, -43.1165) projected
  line L11 (-135.7313, -43.1165) -> (-129.3812, -43.1165) projected
  line L12 (-129.3812, -43.1165) -> (-129.3812, -36.7665) projected
  line L13 (-129.3812, -36.7665) -> (-123.0313, -36.7665) projected
  line L14 (-123.0313, -36.7665) -> (-123.0313, -43.1165) projected
  line L15 (-123.0313, -43.1165) -> (-116.6813, -43.1165) projected
  line L16 (-116.6813, -43.1165) -> (-116.6813, -36.7665) projected
  line L17 (-116.6813, -36.7665) -> (-110.3313, -36.7665) projected
  line L18 (-110.3313, -36.7665) -> (-110.3313, -43.1165) projected
  line L19 (-110.3313, -43.1165) -> (-103.9813, -43.1165) projected
  line L20 (-103.9813, -43.1165) -> (-103.9813, -36.7665) projected
  line L21 (-103.9813, -36.7665) -> (-97.6313, -36.7665) projected
  line L22 (-97.6313, -36.7665) -> (-97.6313, -43.1165) projected
  line L23 (-97.6313, -43.1165) -> (-91.2812, -43.1165) projected
  line L24 (-91.2812, -43.1165) -> (-91.2812, -36.7665) projected
  line L25 (-91.2812, -36.7665) -> (-84.9313, -36.7665) projected
  line L26 (-84.9313, -36.7665) -> (-84.9313, -43.1165) projected
  line L27 (-84.9313, -43.1165) -> (-78.5813, -43.1165) projected
  line L28 (-78.5813, -43.1165) -> (-78.5813, -36.7665) projected
  line L29 (-78.5813, -36.7665) -> (-72.2313, -36.7665) projected
  line L30 (-72.2313, -36.7665) -> (-72.2313, -43.1165) projected
  line L31 (-72.2313, -43.1165) -> (-65.8813, -43.1165) projected
  line L32 (-65.8813, -43.1165) -> (-65.8813, -36.7665) projected
  line L33 (-38.1, 44.45) -> (38.1, 44.45) construction
  line L34 (0, 135.6878) -> (0, 44.45) construction
  constraints: 4 end point
ref_plane "Work Plane5" through (0, 135.6878, 6.35) normal (1, 0, 0) x (0, -1, 0)
mirror "Mirror1" about plane through (0, 135.6878, 6.35) normal (1, 0, 0) of "Extrusion3"
ref_plane "Work Plane6" through (-93.1308, 12.7, 3.175) normal (0, -1, 0) x (0, 0, -1)
ref_plane "Work Plane7" through (-93.1308, 19.05, 3.175) normal (0, 1, 0) x (0, 0, 1)
sketch "Sketch7" plane through (-93.1308, 19.05, 3.175) normal (0, 1, 0) x (0, 0, 1)
  line L0 (3.175, -11.6295) -> (3.175, -49.7295) projected
  line L1 (25.4, 33.5996) -> (3.175, -49.7295) projected
  line L2 (-25.4, 33.5996) -> (25.4, 33.5996) projected
  line L3 (-3.175, -49.7295) -> (-25.4, 33.5996) projected
  line L4 (-3.175, -49.7295) -> (-3.175, -11.6295) projected
  line L5 (-3.175, -11.6295) -> (3.175, -11.6295) projected
  line L6 (3.175, 33.5996) -> (3.175, -11.6295)
  line L7 (3.175, -11.6295) -> (-3.175, -11.6295)
  line L8 (-3.175, -11.6295) -> (-3.175, 33.5996)
  line L9 (-3.175, 33.5996) -> (3.175, 33.5996)
  point P0 (-3.175, 93.1308)
  constraints: 8 end point
extrude "Extrusion4" cut sketch "Sketch7" against normal blind 6.35
mirror "Mirror2" about plane through (0, 135.6878, 6.35) normal (1, 0, 0) of "Extrusion4"